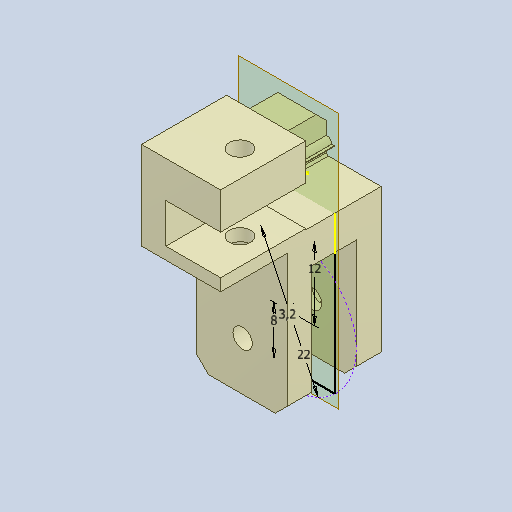
# Autodesk Inventor part: ограничитель
Saved by Autodesk Inventor 2023.1 (Build 271208000, 208)
## iProperties
Created: 2025-12-22
Part Number: ограничитель
Material: Полипропилен
Document SubType Name: Modeling
Designer: DELL
Density: 0.899 g/cm^3
Appearance: Гладкий — пепельный
Author: DELL
Autodesk Inventor part; units mm, degrees
ref_plane "YZ Plane" through (0, 0, 0) normal (1, 0, 0) x (0, 1, 0)
ref_plane "XZ Plane" through (0, 0, 0) normal (0, 1, 0) x (-1, 0, 0)
ref_plane "XY Plane" through (0, 0, 0) normal (0, 0, 1) x (1, 0, 0)
sketch "Эскиз2" plane through (0, 0, 0) normal (0, 0, 1) x (1, 0, 0)
  line L0 (-4.5, 3.25) -> (4.5, 3.25)
  line L1 (4.5, 3.25) -> (4.5, -3.25)
  line L2 (4.5, -3.25) -> (-4.5, -3.25)
  line L3 (-4.5, -3.25) -> (-4.5, 3.25)
  line L4 (-4.5, 3.25) -> (4.5, -3.25) construction
  line L5 (4.5, 3.25) -> (-4.5, -3.25) construction
  line L6 (8.5, 9.25) -> (4.5, 9.25) construction
  line L7 (-8.5, 9.25) -> (-8.5, -5.25)
  line L8 (-8.5, -5.25) -> (4.5, -5.25)
  line L9 (8.5, -5.25) -> (8.5, 9.25) construction
  line L10 (4.5, 3.25) -> (4.5, 9.25)
  line L11 (4.5, -3.25) -> (4.5, -5.25)
  line L12 (4.5, 9.25) -> (-8.5, 9.25)
  line L13 (4.5, -5.25) -> (8.5, -5.25) construction
  point P0 (0, 0)
  dimension "d0" = 9
  dimension "d1" = 6.5
  dimension "d2" = 6
  constraints: 28 end point, 7 parallel, 7 perpendicular, 2 midpoint, 1 horizontal
  measures "d0" distance of L1.end L2.end
  measures "d1" distance of L0.end L1.end
  measures "d2" distance between parallel lines of L0 L6
extrude "Выдавливание1" add sketch "Эскиз2" along normal blind 14 contours L3 L2 L11 L8 L7 L12 L10 L0
sketch "Эскиз3" plane through (-8.5, 9.25, 0) normal (0, 1, 0) x (1, 0, 0)
  line L0 (13, 0) -> (0, 0) construction
  circle A0 centre (8.695, -6.5) radius 1.75
  line L1 (13, 0) -> (13, -14) projected
  point P0 (8.5, 0)
  dimension "d5" = 3.5
  dimension "d9" = 4.305
  constraints: 1 centre point
  measures "d5" diameter of A0
  measures "d9" distance from line of L1 A0.centre
extrude "Выдавливание2" cut sketch "Эскиз3" against normal blind 20
sketch "Эскиз4" plane through (0, 0, 0) normal (0, 0, -1) x (-1, 0, 0)
  line L0 (2.9551, -1.2625) -> (2.9551, -1.7625) construction
  line L1 (2.9551, -1.7625) -> (3.4551, -1.7625) construction
  arc A0 (3.4551, -1.7625) -> (4.305, -2.445) centre (4.405, -1.45) ccw construction
  line L2 (4.305, -2.445) -> (4.305, -3.05) construction
  line L3 (4.305, -3.05) -> (4.105, -3.25) construction
  line L4 (4.105, -3.25) -> (-4.495, -3.25) construction
  line L5 (-4.495, -3.25) -> (-4.695, -3.05) construction
  line L6 (-4.695, -3.05) -> (-4.695, -2.445) construction
  arc A1 (-4.695, -2.445) -> (-3.8451, -1.7625) centre (-4.795, -1.45) ccw construction
  line L7 (-3.8451, -1.7625) -> (-3.3451, -1.7625) construction
  line L8 (-3.3451, -1.7625) -> (-3.3451, -1.2625) construction
  line L9 (-3.3451, -1.2625) -> (-3.8127, -1.2625) construction
  arc A2 (-3.8127, -1.2625) -> (-4.695, -0.455) centre (-4.795, -1.45) ccw construction
  line L10 (-4.695, -0.455) -> (-4.695, 3.05) construction
  line L11 (-4.695, 3.05) -> (-4.495, 3.25) construction
  line L12 (-4.495, 3.25) -> (4.105, 3.25) construction
  line L13 (4.105, 3.25) -> (4.305, 3.05) construction
  line L14 (4.305, 3.05) -> (4.305, -0.455) construction
  arc A3 (4.305, -0.455) -> (3.4227, -1.2625) centre (4.405, -1.45) ccw construction
  line L15 (3.4227, -1.2625) -> (2.9551, -1.2625) construction
  line L16 (4.1878, 3.45) -> (-4.5778, 3.45) construction
  line L17 (-4.5778, 3.45) -> (-4.895, 3.1328) construction
  line L18 (-4.895, 3.1328) -> (-4.895, -0.6563) construction
  arc A4 (-3.9951, -1.4625) -> (-4.895, -0.6563) centre (-4.795, -1.45) ccw construction
  line L19 (-3.9951, -1.4625) -> (-3.5451, -1.4625) construction
  line L20 (-3.5451, -1.4625) -> (-3.5451, -1.5625) construction
  line L21 (-3.5451, -1.5625) -> (-4.0029, -1.5625) construction
  arc A5 (-4.895, -2.2437) -> (-4.0029, -1.5625) centre (-4.795, -1.45) ccw construction
  line L22 (-4.895, -2.2437) -> (-4.895, -3.1328) construction
  line L23 (-4.895, -3.1328) -> (-4.5778, -3.45) construction
  line L24 (-4.5, -3.45) -> (4.1878, -3.45)
  line L25 (4.1878, -3.45) -> (4.505, -3.1328)
  line L26 (4.505, -3.1328) -> (4.505, -2.2437)
  arc A6 (3.6129, -1.5625) -> (4.505, -2.2437) centre (4.405, -1.45) ccw
  line L27 (3.6129, -1.5625) -> (3.1551, -1.5625)
  line L28 (3.1551, -1.5625) -> (3.1551, -1.4625)
  line L29 (3.1551, -1.4625) -> (3.6051, -1.4625)
  arc A7 (4.505, -0.6563) -> (3.6051, -1.4625) centre (4.405, -1.45) ccw
  line L30 (4.505, -0.6563) -> (4.505, 3.1328)
  line L31 (4.505, 3.1328) -> (4.1878, 3.45)
  line L32 (4.1878, 3.45) -> (8.5, 3.45)
  line L33 (8.5, 9.25) -> (8.5, -5.25) projected
  line L34 (-4.5, -5.25) -> (-4.5, -3.25) projected
  line L35 (-4.5, -3.45) -> (-4.5, -29.05)
  line L36 (-4.5, -29.05) -> (10.5, -29.05)
  line L37 (10.5, -29.05) -> (10.5, 3.45)
  line L38 (10.5, 3.45) -> (8.5, 3.45)
  point P0 (0, 0)
  dimension "d10" = 0.2
  dimension "d12" = 4.3122
  dimension "d13" = 15
  constraints: 74 end point, 16 point on circle, 8 centre point, 8 horizontal, 6 vertical, 2 perpendicular, 2 point on line, 1 collinear, 49 other
  measures "d10" distance between parallel lines of L12 L16
  measures "d12" distance of L16.start L32.end
  measures "d13" distance of L35.end L36.end
extrude "Выдавливание3" add sketch "Эскиз4" along normal blind 12.4 and the other way blind 3
chamfer "Фаска1" distance 2 angle 45 1 edges at (-8.5, 3.45, 1.5)
chamfer "Фаска2" distance 2 angle 45 2 edges at (-9.5, 3.45, 0) (-6.3439, 3.45, 0)
chamfer "Фаска3" distance 2 angle 45 2 edges at (-8.5, 4.4499, 3) (-8.5, -0.9, 3)
ref_plane "РабПлоскость1" through (0, 0, -4.7) normal (0, 0, -1) x (-1, 0, 0)
sketch "Эскиз5" plane through (0, 0, -4.7) normal (0, 0, -1) x (-1, 0, 0)
  circle A0 centre (2.8764, -21.05) radius 11 construction
  line L0 (-4.5, -29.05) -> (10.5, -29.05) construction
  circle A1 centre (2.8764, -21.05) radius 1.6
  line L1 (10.5, -29.05) -> (10.5, 3.45) projected
  line L2 (10.5, -29.05) -> (10.5, -9.05)
  line L3 (10.5, -9.05) -> (-4.5, -9.05)
  line L4 (-4.5, -3.45) -> (-4.5, -29.05) projected
  line L5 (-4.5, -9.05) -> (-4.5, -29.05)
  line L6 (-4.5, -29.05) -> (10.5, -29.05)
  point P0 (0, 0)
  dimension "d27" = 22
  dimension "d28" = 8
  dimension "d29" = 3.2
  dimension "d30" = 12
  constraints: 8 end point, 2 centre point, 2 perpendicular, 2 point on line, 1 coincident, 1 collinear
  measures "d27" diameter of A0
  measures "d28" distance from line of A0.centre L0
  measures "d29" diameter of A1
  measures "d30" distance from line of L3 A1.centre
extrude "Выдавливание4" cut sketch "Эскиз5" along normal mid plane 7.4
extrude "Выдавливание5" cut sketch "Эскиз5" along normal mid plane 20 contours A1
sketch "Эскиз6" plane through (0, 0, -12.4) normal (0, 0, -1) x (-1, 0, 0)
  circle A0 centre (2.8764, -21.05) radius 1.6 construction
  circle A1 centre (2.8764, -21.05) radius 1.6 projected
  line L0 (4.5507, -23.95) -> (1.2021, -23.95)
  line L1 (1.2021, -23.95) -> (-0.4722, -21.05)
  line L2 (-0.4722, -21.05) -> (1.2021, -18.15)
  line L3 (1.2021, -18.15) -> (4.5507, -18.15)
  line L4 (4.5507, -18.15) -> (6.2251, -21.05)
  line L5 (6.2251, -21.05) -> (4.5507, -23.95)
  line L6 (-4.5, -29.05) -> (10.5, -29.05) projected
  point P0 (0, 0)
  dimension "d35" = 5.8
  constraints: 12 end point, 1 coincident, 1 parallel, 13 other
  measures "d35" distance between parallel lines of L0 L3
extrude "Выдавливание6" cut sketch "Эскиз6" against normal blind 2.4
chamfer "Фаска4" distance 2 angle 45 5 edges at (-10.5, -29.05, -10.4) (-10.5, -29.05, 1) (4.5, -29.05, 1) (4.5, -29.05, -10.4) (-7.3439, 3.45, -12.4)
